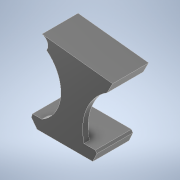
# Autodesk Inventor part: Pieza2_Carcasa
Saved by Autodesk Inventor 2022 (Build 260153000, 153)
## iProperties
Created: 2022-11-06
Part Number: Pieza2_Carcasa
Material: Resina acetálica, negra
Document SubType Name: Modeling
Designer: Mauricio Guerrero
Density: 1.425 g/cm^3
Appearance: Suave - Negro
Author: Mauricio Guerrero
## iProperties of the stored document Pieza2_Carcasa_3DPrint.ipt
Created: 2022-11-06
Part Number: Pieza2_Carcasa_3DPrint
Material: Genérico
Document SubType Name: Modeling
Designer: Mauricio Guerrero
Density: 1 g/cm^3
Appearance: Valor por defecto
Author: Mauricio Guerrero
Autodesk Inventor part; units mm, degrees
ref_plane "YZ Plane" through (0, 0, 0) normal (1, 0, 0) x (0, 1, 0)
ref_plane "XZ Plane" through (0, 0, 0) normal (0, 1, 0) x (-1, 0, 0)
ref_plane "XY Plane" through (0, 0, 0) normal (0, 0, 1) x (1, 0, 0)
sketch "Boceto1" plane through (0, 0, 0) normal (0, 0, 1) x (1, 0, 0)
  line L0 (19.6774, 4.2368) -> (8.7831, 5.4266)
  line L1 (17.5677, -5.7575) -> (6.2503, -5.7575)
  line L2 (19.6774, 4.2368) -> (8.7831, 5.4266)
  line L3 (8.7831, 5.4266) -> (19.6774, 4.2368)
  line L4 (17.3447, -5.7575) -> (8.5436, -5.7575)
  line L5 (7.079, -7.7575) -> (17.1134, -7.7575)
  line L6 (7.7997, 7.5459) -> (20.665, 6.1409)
  line L7 (19.6774, 4.2368) -> (20.665, 6.1409)
  line L8 (7.079, -7.7575) -> (6.0556, -6.3899)
  line L9 (6.0556, -6.3899) -> (6.2503, -5.7575)
  line L10 (17.1134, -7.7575) -> (17.8267, -6.1873)
  line L11 (17.8267, -6.1873) -> (17.5677, -5.7575)
  arc A0 (8.7831, 5.4266) -> (7.7997, 7.5459) centre (7.7394, 6.2301) ccw
  point P0 (7.9645, 7.5279)
  dimension "d9" = 2
  dimension "d10" = 2
  constraints: 24 end point, 2 horizontal, 2 point on circle, 1 centre point, 1 collinear, 1 other
  measures "d9" distance between parallel lines of L0 L6
  measures "d10" distance between parallel lines of L1 L5
extrude "Extrusión1" add sketch "Boceto1" along normal blind 6.5
sketch "Boceto3" plane through (0, 0, 6.5) normal (0, 0, 1) x (1, 0, 0)
  line L0 (17.5677, -5.7575) -> (6.2503, -5.7575) projected
  line L1 (7.9375, -5.7575) -> (15.5213, -5.7575)
  line L2 (8.7831, 5.4266) -> (19.6774, 4.2368) projected
  line L3 (8.7748, 5.433) -> (19.685, 4.2415)
  arc A0 (7.9375, -5.7575) -> (8.7831, 5.4266) centre (4.6391, 0.1159) ccw
  arc A1 (19.6774, 4.2368) -> (15.5213, -5.7575) centre (24.5927, -3.6684) ccw
  line L4 (15.5213, -5.7575) -> (7.9375, -5.7575)
  line L5 (17.5677, -5.7575) -> (6.2503, -5.7575) projected
  point P0 (0, 0)
  point P1 (18.2329, -5.7575)
  point P2 (5.3085, -5.7575)
  point P3 (8.358, 5.473)
  point P4 (20.8396, 4.1099)
  point P5 (8.7666, 5.4284)
  constraints: 6 end point, 6 point on circle, 2 centre point, 2 point on line, 1 collinear, 1 parallel
extrude "Extrusión3" add sketch "Boceto3" against normal blind 1
